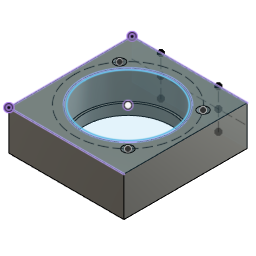
FrontCenterRodSupportAssembly v5 (Autodesk Fusion 360 archive; units mm, degrees)
design "CenterRodBearingSupport" references "tormach 770mx"
Autodesk Fusion 360 part; units mm, degrees
sketch "Sketch1" plane through (0, 0, 0) normal (0, 1, 0) x (1, 0, 0)
  line L0 (60, 0) -> (60, -30)
  line L1 (0, -15) -> (60, -15) construction
  line L2 (32, 0) -> (32, -30) construction
  line L3 (46, 0) -> (46, -30) construction
  line L4 (60, 0) -> (32, 0)
  line L5 (32, 0) -> (32, -30)
  line L6 (32, -30) -> (60, -30)
  line L7 (60, -30) -> (60, 0)
  dimension "d39" = 14
  dimension "d40" = 28
  dimension "d42" = 30
  constraint vertical L0
  constraint midpoint L0 L1.end
  constraint horizontal L4
  constraint vertical L5
  constraint horizontal L6
  constraint vertical L7
  measures "d39" distance of L0 L3
  measures "d40" distance of L0 L2
  measures "d42" distance of L0.start L0.end
extrude "Extrude1" add sketch "Sketch1" along normal blind 9.6
sketch "Sketch2" plane through (0, 9.6, 0) normal (0, 1, 0) x (-1, 0, 0)
  line L0 (-60, 30) -> (-60, 0)
  circle A0 centre (-46, 15) radius 11.05
  circle A1 centre (-46, 15) radius 10.55
  line L1 (-60, 0) -> (-32, 0)
  line L2 (-32, 0) -> (-32, 30)
  line L3 (-32, 30) -> (-60, 30)
  dimension "d15" = 22.1
  dimension "d16" = 21.1
  constraint concentric A0 A1
  measures "d15" diameter of A0
  measures "d16" diameter of A1
extrude "Extrude2" cut sketch "Sketch2" against normal blind 7 contours A0
extrude "Extrude3" cut 1 faces at (43.0944, 9.6, 14.0673) along direction (0, 1, 0) through all and the other way through all
sketch "Sketch3" plane through (0, 9.6, 0) normal (0, 1, 0) x (-1, 0, 0)
  line L0 (-60, 30) -> (-60, 0)
  circle A0 centre (-46, 15) radius 13 construction
  line L1 (-32, 30) -> (-60, 30)
  line L2 (-60, 0) -> (-32, 0)
  line L3 (-32, 0) -> (-32, 30)
  circle A1 centre (-46, 15) radius 11.05
  point P0 (-35.8444, 6.8844)
  point P1 (-55.1828, 24.202)
  point P2 (-56.1556, 6.8844)
  dimension "d30" = 26
  constraint concentric A0 A1
  constraint coincident A0 P0
  constraint coincident A0 P1
  constraint coincident A0 P2
  measures "d30" diameter of A0
hole "Hole1" at (35.8444, 9.6, 6.8844) direction (0, -1, 0) diameter 2.5 end through all
hole "Hole2" at (56.1556, 9.6, 6.8844) direction (0, -1, 0) diameter 2.5 end through all
hole "Hole3" at (55.1828, 9.6, 24.202) direction (0, -1, 0) diameter 2.5 end through all
sketch "Sketch4" plane through (0, 0, 0) normal (0, 0, -1) x (-1, 0, 0)
  line L0 (-60, 0) -> (-32, 0)
  line L1 (-32, 0) -> (-32, 9.6)
  line L2 (-32, 9.6) -> (-60, 9.6)
  line L3 (-60, 9.6) -> (-60, 0)
  line L4 (-32, 4.8) -> (-60, 4.8) construction
  line L5 (-39, 0) -> (-39, 9.6) construction
  line L6 (-53, 0) -> (-53, 9.6) construction
  point P0 (-39, 4.8)
  point P1 (-53, 4.8)
  dimension "d43" = 14
  dimension "d44" = 7
  constraint midpoint L1 L4.start
  constraint midpoint L3 L4.end
  constraint coincident L0 L5.start
  constraint coincident L2 L5.end
  constraint perpendicular L2 L5
  constraint coincident L0 L6.start
  constraint coincident L2 L6.end
  constraint perpendicular L2 L6
  constraint midpoint L5 P0
  constraint midpoint L6 P1
  measures "d43" distance of L5 L6
  measures "d44" distance of L1 L5
hole "Hole4" at (39, 4.8, 0) direction (0, 0, 1) diameter 3.3 depth 4 tip angle 118
hole "Hole5" at (53, 4.8, 0) direction (0, 0, 1) diameter 3.3 depth 4 tip angle 118
